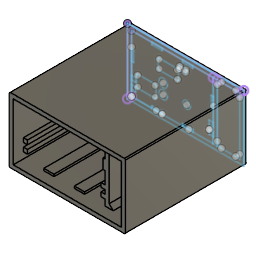
DD-boitier-V5 (Autodesk Fusion 360 design; units mm, degrees)
part number: 2025-12-19-14-32-53-043
Autodesk Fusion 360 part; units mm, degrees
sketch "Esquisse1" plane through (0, 0, 0) normal (0, 1, 0) x (1, 0, 0)
  line L0 (0, -28) -> (40, -28)
  line L1 (40, -28) -> (40, 0)
  line L2 (40, 0) -> (42, 0)
  line L3 (42, 0) -> (42, -28)
  line L4 (42, -28) -> (40, -28)
  line L5 (40, -28) -> (40, 0)
  line L6 (42, 0) -> (53, 0)
  line L7 (53, 0) -> (53, -28)
  line L8 (53, -28) -> (42, -28)
  line L9 (42, -28) -> (42, 0)
  line L10 (12, 0) -> (15, 0)
  line L11 (25, 0) -> (28, 0)
  line L12 (10, -28) -> (15, -28)
  line L13 (15, -28) -> (15, -27)
  line L14 (15, -27) -> (10, -27)
  line L15 (10, -27) -> (10, -28)
  line L16 (30, -28) -> (25, -28)
  line L17 (25, -28) -> (25, -27)
  line L18 (25, -27) -> (30, -27)
  line L19 (30, -27) -> (30, -28)
  line L20 (0, -3) -> (2, -3)
  line L21 (2, -3) -> (2, -5)
  line L22 (2, -5) -> (0, -5)
  line L23 (0, -5) -> (0, -3)
  line L24 (40, -3) -> (38, -3)
  line L25 (38, -3) -> (38, -5)
  line L26 (38, -5) -> (40, -5)
  line L27 (40, -5) -> (40, -3)
  line L28 (40, -7) -> (38, -7)
  line L29 (38, -7) -> (38, -9)
  line L30 (38, -9) -> (40, -9)
  line L31 (40, -9) -> (40, -7)
  line L32 (2.9548, -4.9937) -> (11.5266, -4.9937)
  line L33 (12.0266, -5.4937) -> (12.0266, -10.4824)
  line L34 (11.5266, -10.9824) -> (2.9548, -10.9824)
  line L35 (2.4548, -10.4824) -> (2.4548, -5.4937)
  circle A0 centre (27, -10) radius 1.75
  circle A1 centre (15.5, -8.5) radius 2
  circle A2 centre (15.5, -13.5) radius 2
  line L36 (0, 0) -> (40, 0)
  line L37 (0, 0) -> (0, -28)
  line L38 (0, -7) -> (2, -7)
  line L39 (2, -7) -> (2, -9)
  line L40 (2, -9) -> (0, -9)
  line L41 (0, -9) -> (0, -7)
  line L42 (-2, -30) -> (55, -30)
  line L43 (55, -30) -> (55, 2)
  line L44 (55, 2) -> (-2, 2)
  line L45 (-2, 2) -> (-2, -30)
  line L46 (0, 0) -> (15, 0)
  line L47 (13.5, -18) -> (22.531, -18)
  line L48 (23.031, -18.5) -> (23.031, -22.5239)
  line L49 (22.531, -23.0239) -> (13.5, -23.0239)
  line L50 (13, -22.5239) -> (13, -18.5)
  line L51 (0, -20) -> (1, -20)
  line L52 (1, -20) -> (1, -15)
  line L53 (1, -15) -> (0, -15)
  line L54 (0, -15) -> (0, -20)
  line L55 (40, -16) -> (40, -20)
  line L56 (44, -28) -> (42, -26)
  line L57 (51, -28) -> (53, -26)
  line L58 (53, -2) -> (51, 0)
  line L59 (44, 0) -> (42, -2)
  line L60 (10, 0) -> (15, 0)
  line L61 (15, 0) -> (15, -1)
  line L62 (15, -1) -> (10, -1)
  line L63 (10, -1) -> (10, 0)
  line L64 (25, 0) -> (30, 0)
  line L65 (30, 0) -> (30, -1)
  line L66 (30, -1) -> (25, -1)
  line L67 (25, -1) -> (25, 0)
  line L68 (40, -20) -> (39, -20)
  line L69 (39, -20) -> (39, -15)
  line L70 (39, -15) -> (40, -15)
  line L71 (40, -15) -> (40, -20)
  line L72 (0, -21) -> (0, 0)
  line L73 (27, -23.5239) -> (27, -24.5)
  line L74 (26.5, -25) -> (23.5232, -25)
  arc A3 (11.5266, -10.9824) -> (12.0266, -10.4824) centre (11.5266, -10.4824) ccw
  arc A4 (2.4548, -10.4824) -> (2.9548, -10.9824) centre (2.9548, -10.4824) ccw
  arc A5 (2.9548, -4.9937) -> (2.4548, -5.4937) centre (2.9548, -5.4937) ccw
  arc A6 (12.0266, -5.4937) -> (11.5266, -4.9937) centre (11.5266, -5.4937) ccw
  arc A7 (13.5, -18) -> (13, -18.5) centre (13.5, -18.5) ccw
  arc A8 (13, -22.5239) -> (13.5, -23.0239) centre (13.5, -22.5239) ccw
  arc A9 (23.031, -18.5) -> (22.531, -18) centre (22.531, -18.5) ccw
  arc A10 (22.531, -23.0239) -> (23.031, -22.5239) centre (22.531, -22.5239) ccw
  line L75 (26.5, -23.0239) -> (23.5079, -23.0239)
  line L76 (23.008, -23.5318) -> (23.0233, -24.5078)
  arc A11 (23.5079, -23.0239) -> (23.008, -23.5318) centre (23.5079, -23.5239) ccw
  arc A12 (27, -23.5239) -> (26.5, -23.0239) centre (26.5, -23.5239) ccw
  arc A13 (26.5, -25) -> (27, -24.5) centre (26.5, -24.5) ccw
  arc A14 (23.0233, -24.5078) -> (23.5232, -25) centre (23.5232, -24.5) ccw
  dimension "d90" = 0.5
  constraint horizontal L0
  constraint vertical L1
  constraint horizontal L2
  constraint vertical L3
  constraint horizontal L4
  constraint vertical L5
  constraint horizontal L6
  constraint vertical L7
  constraint horizontal L8
  constraint vertical L9
  constraint horizontal L10
  constraint horizontal L11
  constraint horizontal L12
  constraint vertical L13
  constraint horizontal L14
  constraint vertical L15
  constraint horizontal L16
  constraint vertical L17
  constraint horizontal L18
  constraint vertical L19
  constraint horizontal L20
  constraint vertical L21
  constraint horizontal L22
  constraint vertical L23
  constraint horizontal L24
  constraint vertical L25
  constraint horizontal L26
  constraint vertical L27
  constraint horizontal L28
  constraint vertical L29
  constraint horizontal L30
  constraint vertical L31
  constraint horizontal L32
  constraint vertical L33
  constraint horizontal L34
  constraint vertical L35
  constraint perpendicular L1 L36
  constraint perpendicular L0 L37
  constraint horizontal L38
  constraint vertical L39
  constraint horizontal L40
  constraint vertical L41
  constraint horizontal L42
  constraint vertical L43
  constraint horizontal L44
  constraint vertical L45
  constraint horizontal L46
  constraint horizontal L47
  constraint vertical L48
  constraint horizontal L49
  constraint vertical L50
  constraint horizontal L51
  constraint vertical L52
  constraint horizontal L53
  constraint vertical L54
  constraint vertical L55
  constraint perpendicular L56 L57
  constraint perpendicular L57 L58
  constraint perpendicular L58 L59
  constraint horizontal L60
  constraint vertical L61
  constraint horizontal L62
  constraint vertical L63
  constraint horizontal L64
  constraint vertical L65
  constraint horizontal L66
  constraint vertical L67
  constraint horizontal L68
  constraint vertical L69
  constraint horizontal L70
  constraint vertical L71
  constraint vertical L72
  constraint vertical L73
  constraint horizontal L74
  constraint tangent L33 A3
  constraint tangent L34 A3
  constraint tangent L34 A4
  constraint tangent L35 A4
  constraint equal A3 A4
  constraint tangent L32 A5
  constraint tangent L35 A5
  constraint equal A3 A5
  constraint tangent L32 A6
  constraint tangent L33 A6
  constraint equal A3 A6
  constraint tangent L47 A7
  constraint tangent L50 A7
  constraint equal A3 A7
  constraint tangent L49 A8
  constraint tangent L50 A8
  constraint equal A3 A8
  constraint tangent L47 A9
  constraint tangent L48 A9
  constraint tangent L48 A10
  constraint tangent L49 A10
  constraint equal A9 A10
  constraint perpendicular L73 L75
  constraint tangent L75 A11
  constraint tangent L76 A11
  constraint tangent L73 A12
  constraint tangent L75 A12
  constraint equal A11 A12
  constraint tangent L73 A13
  constraint tangent L74 A13
  constraint equal A11 A13
  constraint tangent L74 A14
  constraint tangent L76 A14
  constraint equal A11 A14
  measures "d90" radius of A11
sketch "Esquisse2" plane through (0, 0, 0) normal (0, 1, 0) x (1, 0, 0)
sketch "Esquisse3" plane through (0, 0, 0) normal (0, 1, 0) x (1, 0, 0)
  line L0 (-2, -30) -> (55, -30)
  line L1 (-2, 2) -> (-2, -30)
  dimension "d54" = 57
  dimension "d55" = 32
  measures "d54" distance of L0.start L0.end
  measures "d55" distance of L0.start L1.start
sketch "Esquisse4" plane through (0, 0, 0) normal (0, 0, 1) x (1, 0, 0)
sketch "Esquisse5" plane through (0, 0, 0) normal (0, 1, 0) x (1, 0, 0)
  line L0 (-2, 2) -> (-2, -30)
  line L1 (0, 0) -> (0, -28)
  line L2 (-2, -30) -> (55, -30)
  line L3 (0, -28) -> (40, -28)
  line L4 (42, -28) -> (40, -28)
  line L5 (53, -28) -> (42, -28)
  dimension "d80" = 32
  dimension "d81" = 28
  dimension "d82" = 57
  dimension "d83" = 40
  dimension "d84" = 2
  dimension "d85" = 11
  measures "d80" distance of L0.start L0.end
  measures "d81" distance of L1.start L1.end
  measures "d82" distance of L0.end L2.end
  measures "d83" distance of L1.end L3.end
  measures "d84" distance of L4.start L3.end
  measures "d85" distance of L5.start L4.start
extrude "Extrusion18" add sketch "Esquisse1" along normal blind 1.5 contours L0 L1 L5 L13 L14 L15 L17 L18 L19 L20 L21 L22 L24 L25 L26 L28 L29 L30 L36 L37 L38 L39 L40 L46 L51 L52 L53 L61 L62 L63 L65 L66 L67 L68 L69 L70 L72 | L0 L12 L13 L14 L15 | L37 L51 L52 L53 L54 L72 | L0 L16 L17 L18 L19 | L37 L38 L39 L40 L41 L72 | L1 L2 L3 L4 L5 L9 L27 L31 L55 L71 | L1 L5 L55 L68 L69 L70 L71 | L3 L8 L9 L56 | L20 L21 L22 L23 L37 L72 | L3 L6 L7 L8 L9 L56 L57 L58 L59 | L3 L6 L9 L59 | L7 L8 L57 | L1 L5 L28 L29 L30 L31 | L10 L36 L46 L60 L61 L62 L63 | L6 L7 L58 | L1 L5 L24 L25 L26 L27 | L11 L36 L64 L65 L66 L67 | L42 L43 L44 L45 | L73 L74 L75 L76 A11 A12 A13 A14 makes body 1
extrude "Extrusion19" add sketch "Esquisse1" against normal blind 58 separate body contours L42 L43 L44 L45 makes body 2
extrude "Extrusion20" add sketch "Esquisse1" against normal blind 53 separate body contours L0 L12 L13 L14 L15 | L0 L16 L17 L18 L19 | L37 L38 L39 L40 L41 L72 | L1 L5 L55 L68 L69 L70 L71 | L3 L8 L9 L56 | L20 L21 L22 L23 L37 L72 | L3 L6 L9 L59 | L7 L8 L57 | L1 L5 L28 L29 L30 L31 | L10 L36 L46 L60 L61 L62 L63 | L6 L7 L58 | L1 L5 L24 L25 L26 L27 | L11 L36 L64 L65 L66 L67 makes body 3 at (39, -17.6667, 18.3333) makes body 4 at (0, -17.6667, 4.3333) makes body 5 at (52.3333, -17.6667, 1.3333) makes body 6 at (43.3333, -17.6667, 27.3333) makes body 7 at (11.6667, -17.6667, 0) makes body 8 at (38.6667, -17.6667, 9) makes body 9 at (13.3333, -17.6667, 27) makes body 10 at (0, -17.6667, 7.6667) makes body 11 at (43.3333, -35.3333, 0.6667) makes body 12 at (51.6667, -35.3333, 27.3333) makes body 13 at (28.3333, -17.6667, 1) makes body 14 at (38.6667, -17.6667, 5) makes body 15 at (26.6667, -17.6667, 27)
extrude "Extrusion21" add sketch "Esquisse1" along normal blind 1 separate body contours L73 L74 L75 L76 A11 A12 A13 A14 makes body 16
extrude "Extrusion22" cut sketch "Esquisse1" along normal blind 1 contours L73 L74 L75 L76 A11 A12 A13 A14 bodies 1 16
fillet "Congé6" radius 0.5 1 edges at (26.5, 1.5, 30) on bodies 1
fillet "Congé7" radius 0.5 3 edges at (55, 0.5, 30) (55, 1.3536, 29.8536) (55, 1.5, 13.75) on bodies 1
fillet "Congé8" radius 0.5 1 edges at (55, -29, 30) on bodies 2
fillet "Congé9" radius 0.5 1 edges at (55, -29, -2) on bodies 2
fillet "Congé10" radius 0.5 3 edges at (55, 0.5, -2) (54.8536, 1.3536, -2) (26.25, 1.5, -2) on bodies 1
fillet "Congé11" radius 0.5 5 edges at (-2, 0.5, -2) (-2, 1.3536, -1.8536) (-2, 1.5, 14) (-2, 1.3536, 29.8536) (-2, 0.5, 30) on bodies 1
fillet "Congé12" radius 0.5 1 edges at (-2, -29, -2) on bodies 2
fillet "Congé13" radius 0.5 1 edges at (-2, -29, 30) on bodies 2
extrude "Extrusion23" add sketch "Esquisse1" against normal blind 53 contours L1 L2 L3 L4 L5 L9 L27 L31 L55 L71 bodies 1 4 5 7 9 10 12 13 15 2 3 6 8 11 14 16
extrude "Extrusion1" [suppressed]
extrude "Extrusion2" [suppressed]
extrude "Extrusion3" [suppressed]
